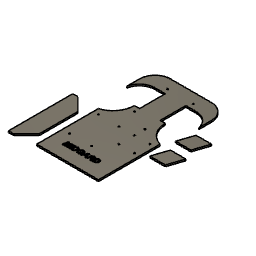
MIDGARD 3d (Autodesk Fusion 360 design; units mm, degrees)
Autodesk Fusion 360 part; units mm, degrees
note: some values were not read from the file. Chosen so that the rebuilt part matches the saved one: which bodies a step acts on.
sketch "Sketch1" plane through (0, 0, 0) normal (0, 1, 0) x (1, 0, 0)
  line L0 (60, 0) -> (60, -120)
  line L1 (60, -120) -> (-60, -120)
  line L2 (-60, -120) -> (-60, 0)
  line L3 (20, 40) -> (20, 90)
  line L4 (-20, 90) -> (-20, 40)
  line L5 (40, 120) -> (-40, 120)
  arc A0 (-40, 120) -> (-70, 90) centre (-40, 90) ccw
  line L6 (-70, 90) -> (-70, 65)
  arc A1 (-40, 90) -> (-70, 65) centre (-40, 59.5) ccw
  arc A2 (70, 90) -> (40, 120) centre (40, 90) ccw
  line L7 (70, 90) -> (70, 65)
  arc A3 (70, 65) -> (70, 66.4639) centre (45.1933, 65.732) ccw
  arc A4 (-60, 0) -> (-30, 40) centre (-71.6667, 40) ccw
  arc A5 (30, 40) -> (60, 0) centre (71.6667, 40) ccw
  arc A6 (70, 65) -> (40, 90) centre (40, 59.5) ccw
  line L8 (30, 40) -> (20, 40)
  line L9 (-20, 40) -> (-30, 40)
  line L10 (-40, 90) -> (-20, 90)
  line L11 (20, 90) -> (40, 90)
  line L12 (-75, -100) -> (-75, -25)
  line L13 (-100, 0) -> (-75, -25)
  line L14 (-75, -100) -> (-100, -125)
  line L15 (80, 50) -> (110, 50)
  line L16 (110, 50) -> (100, 20)
  line L17 (100, 20) -> (70, 20)
  line L18 (70, 20) -> (80, 50)
  line L19 (80, 0) -> (110, 0)
  line L20 (110, 0) -> (100, -30)
  line L21 (70, -30) -> (80, 0)
  line L22 (100, -30) -> (70, -30)
  line L23 (-110, 0) -> (-100, 0)
  line L24 (-100, -125) -> (-110, -125)
  line L25 (-110, -125) -> (-110, 0)
  line L26 (-26.9347, -100.4858) -> (-28.8856, -100.4758)
  line L27 (-28.8856, -100.4758) -> (-29.2041, -92.1179)
  line L28 (-29.2041, -92.1179) -> (-30.8365, -100.4657)
  line L29 (-30.8365, -100.4657) -> (-32.6918, -100.4562)
  line L30 (-32.6918, -100.4562) -> (-30.5531, -90.467)
  line L31 (-30.5531, -90.467) -> (-27.6199, -90.4821)
  line L32 (-27.6199, -90.4821) -> (-27.3491, -97.4891)
  line L33 (-27.3491, -97.4891) -> (-23.9024, -90.5013)
  line L34 (-23.9024, -90.5013) -> (-20.9352, -90.5166)
  line L35 (-20.9352, -90.5166) -> (-23.0808, -100.5056)
  line L36 (-23.0808, -100.5056) -> (-24.9566, -100.496)
  line L37 (-24.9566, -100.496) -> (-22.9426, -92.2116)
  line L38 (-22.9426, -92.2116) -> (-26.9347, -100.4858)
  line L39 (-21.1367, -100.5157) -> (-18.9911, -90.5266)
  line L40 (-18.9911, -90.5266) -> (-16.938, -90.5371)
  line L41 (-16.938, -90.5371) -> (-19.0767, -100.5263)
  line L42 (-19.0767, -100.5263) -> (-21.1367, -100.5157)
  line L43 (-17.1327, -100.5363) -> (-14.9871, -90.5472)
  line L44 (-14.9871, -90.5472) -> (-12.2927, -90.5611)
  spline S0 degree 2 poles (-12.2927, -90.5611) (-11.1672, -90.5669) (-10.8536, -90.6026) knots 0 0 0 1 1 1
  spline S1 degree 2 poles (-10.8536, -90.6026) (-10.2332, -90.6672) (-9.7465, -90.8607) knots 0 0 0 1 1 1
  spline S2 degree 2 poles (-9.7465, -90.8607) (-9.2598, -91.0542) (-8.8625, -91.4007) knots 0 0 0 1 1 1
  spline S3 degree 2 poles (-8.8625, -91.4007) (-8.4652, -91.7472) (-8.1778, -92.233) knots 0 0 0 1 1 1
  spline S4 degree 2 poles (-8.1778, -92.233) (-7.8904, -92.7188) (-7.7368, -93.3506) knots 0 0 0 1 1 1
  spline S5 degree 2 poles (-7.7368, -93.3506) (-7.5831, -93.9824) (-7.587, -94.7327) knots 0 0 0 1 1 1
  spline S6 degree 2 poles (-7.587, -94.7327) (-7.5953, -96.3493) (-8.2191, -97.5978) knots 0 0 0 1 1 1
  spline S7 degree 2 poles (-8.2191, -97.5978) (-8.8428, -98.8463) (-9.7811, -99.5782) knots 0 0 0 1 1 1
  spline S8 degree 2 poles (-9.7811, -99.5782) (-10.5003, -100.1475) (-11.634, -100.4145) knots 0 0 0 1 1 1
  spline S9 degree 2 poles (-11.634, -100.4145) (-12.276, -100.5613) (-13.6061, -100.5544) knots 0 0 0 1 1 1
  line L45 (-13.6061, -100.5544) -> (-17.1327, -100.5363)
  line L46 (-14.7302, -98.9388) -> (-13.6865, -98.9442)
  spline S10 degree 2 poles (-13.6865, -98.9442) (-12.5542, -98.95) (-12.0453, -98.8128) knots 0 0 0 1 1 1
  spline S11 degree 2 poles (-12.0453, -98.8128) (-11.5364, -98.6756) (-11.1115, -98.2958) knots 0 0 0 1 1 1
  spline S12 degree 2 poles (-11.1115, -98.2958) (-10.5016, -97.7464) (-10.0808, -96.8277) knots 0 0 0 1 1 1
  spline S13 degree 2 poles (-10.0808, -96.8277) (-9.6599, -95.9089) (-9.6535, -94.6607) knots 0 0 0 1 1 1
  spline S14 degree 2 poles (-9.6535, -94.6607) (-9.648, -93.5966) (-9.9897, -93.0593) knots 0 0 0 1 1 1
  spline S15 degree 2 poles (-9.9897, -93.0593) (-10.3314, -92.5221) (-10.8353, -92.3421) knots 0 0 0 1 1 1
  spline S16 degree 2 poles (-10.8353, -92.3421) (-11.1894, -92.2175) (-12.0966, -92.2128) knots 0 0 0 1 1 1
  line L47 (-12.0966, -92.2128) -> (-13.2903, -92.2067)
  line L48 (-13.2903, -92.2067) -> (-14.7302, -98.9388)
  line L49 (-1.4847, -95.2757) -> (2.99, -95.2988)
  line L50 (2.99, -95.2988) -> (2.0675, -99.5847)
  spline S17 degree 2 poles (2.0675, -99.5847) (1.2737, -100.0922) (0.1225, -100.4409) knots 0 0 0 1 1 1
  spline S18 degree 2 poles (0.1225, -100.4409) (-1.0287, -100.7897) (-2.2224, -100.7836) knots 0 0 0 1 1 1
  spline S19 degree 2 poles (-2.2224, -100.7836) (-4.0778, -100.774) (-5.0626, -99.9299) knots 0 0 0 1 1 1
  spline S20 degree 2 poles (-5.0626, -99.9299) (-6.4073, -98.777) (-6.3961, -96.6011) knots 0 0 0 1 1 1
  spline S21 degree 2 poles (-6.3961, -96.6011) (-6.3885, -95.1413) (-5.8018, -93.8074) knots 0 0 0 1 1 1
  spline S22 degree 2 poles (-5.8018, -93.8074) (-5.0978, -92.2011) (-3.8108, -91.321) knots 0 0 0 1 1 1
  spline S23 degree 2 poles (-3.8108, -91.321) (-2.5239, -90.4408) (-0.7913, -90.4498) knots 0 0 0 1 1 1
  spline S24 degree 2 poles (-0.7913, -90.4498) (0.9413, -90.4587) (1.9842, -91.269) knots 0 0 0 1 1 1
  spline S25 degree 2 poles (1.9842, -91.269) (3.0271, -92.0793) (3.3602, -93.6226) knots 0 0 0 1 1 1
  line L51 (3.3602, -93.6226) -> (1.4423, -93.831)
  spline S26 degree 2 poles (1.4423, -93.831) (1.1943, -92.9839) (0.6338, -92.5513) knots 0 0 0 1 1 1
  spline S27 degree 2 poles (0.6338, -92.5513) (0.0732, -92.1186) (-0.7794, -92.1142) knots 0 0 0 1 1 1
  spline S28 degree 2 poles (-0.7794, -92.1142) (-1.7753, -92.1091) (-2.6102, -92.6232) knots 0 0 0 1 1 1
  spline S29 degree 2 poles (-2.6102, -92.6232) (-3.445, -93.1374) (-3.9213, -94.2195) knots 0 0 0 1 1 1
  spline S30 degree 2 poles (-3.9213, -94.2195) (-4.3975, -95.3016) (-4.4041, -96.584) knots 0 0 0 1 1 1
  spline S31 degree 2 poles (-4.4041, -96.584) (-4.4106, -97.8459) (-3.8408, -98.4526) knots 0 0 0 1 1 1
  spline S32 degree 2 poles (-3.8408, -98.4526) (-3.2709, -99.0592) (-2.1658, -99.0649) knots 0 0 0 1 1 1
  spline S33 degree 2 poles (-2.1658, -99.0649) (-1.5042, -99.0683) (-0.8075, -98.8843) knots 0 0 0 1 1 1
  spline S34 degree 2 poles (-0.8075, -98.8843) (-0.1107, -98.7003) (0.3954, -98.4437) knots 0 0 0 1 1 1
  line L52 (0.3954, -98.4437) -> (0.71, -96.9583)
  line L53 (0.71, -96.9583) -> (-1.8411, -96.9451)
  line L54 (-1.8411, -96.9451) -> (-1.4847, -95.2757)
  line L55 (10.3476, -98.4677) -> (6.3845, -98.4472)
  line L56 (6.3845, -98.4472) -> (5.1726, -100.6511)
  line L57 (5.1726, -100.6511) -> (3.058, -100.6402)
  line L58 (3.058, -100.6402) -> (8.7643, -90.6695)
  line L59 (8.7643, -90.6695) -> (11.0494, -90.6813)
  line L60 (11.0494, -90.6813) -> (12.6213, -100.6895)
  line L61 (12.6213, -100.6895) -> (10.6705, -100.6794)
  line L62 (10.6705, -100.6794) -> (10.3476, -98.4677)
  line L63 (10.1038, -96.802) -> (9.5447, -92.7745)
  line L64 (9.5447, -92.7745) -> (7.1093, -96.7866)
  line L65 (7.1093, -96.7866) -> (10.1038, -96.802)
  line L66 (15.9774, -100.7068) -> (13.9174, -100.6962)
  line L67 (13.9174, -100.6962) -> (16.063, -90.7071)
  line L68 (16.063, -90.7071) -> (20.5036, -90.7299)
  spline S35 degree 2 poles (20.5036, -90.7299) (21.6495, -90.7358) (22.2861, -90.9745) knots 0 0 0 1 1 1
  spline S36 degree 2 poles (22.2861, -90.9745) (22.9227, -91.2131) (23.3117, -91.8426) knots 0 0 0 1 1 1
  spline S37 degree 2 poles (23.3117, -91.8426) (23.7006, -92.4722) (23.696, -93.3658) knots 0 0 0 1 1 1
  spline S38 degree 2 poles (23.696, -93.3658) (23.6895, -94.6414) (22.9212, -95.4662) knots 0 0 0 1 1 1
  spline S39 degree 2 poles (22.9212, -95.4662) (22.153, -96.291) (20.6036, -96.4809) knots 0 0 0 1 1 1
  spline S40 degree 2 poles (20.6036, -96.4809) (20.9974, -96.8376) (21.3423, -97.4192) knots 0 0 0 1 1 1
  spline S41 degree 2 poles (21.3423, -97.4192) (22.0252, -98.596) (22.86, -100.7422) knots 0 0 0 1 1 1
  line L69 (22.86, -100.7422) -> (20.6499, -100.7308)
  spline S42 degree 2 poles (20.6499, -100.7308) (20.3882, -99.8836) (19.6198, -98.0857) knots 0 0 0 1 1 1
  spline S43 degree 2 poles (19.6198, -98.0857) (19.2019, -97.1149) (18.7262, -96.7782) knots 0 0 0 1 1 1
  spline S44 degree 2 poles (18.7262, -96.7782) (18.4339, -96.5788) (17.704, -96.5751) knots 0 0 0 1 1 1
  line L70 (17.704, -96.5751) -> (16.865, -96.5708)
  line L71 (16.865, -96.5708) -> (15.9774, -100.7068)
  line L72 (17.1865, -95.0717) -> (18.2779, -95.0773)
  spline S45 degree 2 poles (18.2779, -95.0773) (19.9354, -95.0859) (20.4787, -94.8909) knots 0 0 0 1 1 1
  spline S46 degree 2 poles (20.4787, -94.8909) (21.022, -94.6958) (21.3312, -94.2745) knots 0 0 0 1 1 1
  spline S47 degree 2 poles (21.3312, -94.2745) (21.6403, -93.8532) (21.6427, -93.3893) knots 0 0 0 1 1 1
  spline S48 degree 2 poles (21.6427, -93.3893) (21.6455, -92.8436) (21.2035, -92.5685) knots 0 0 0 1 1 1
  spline S49 degree 2 poles (21.2035, -92.5685) (20.9315, -92.4034) (20.0243, -92.3987) knots 0 0 0 1 1 1
  line L73 (20.0243, -92.3987) -> (17.7597, -92.3871)
  line L74 (17.7597, -92.3871) -> (17.1865, -95.0717)
  line L75 (23.9991, -100.7481) -> (26.1447, -90.759)
  line L76 (26.1447, -90.759) -> (28.8391, -90.7729)
  spline S50 degree 2 poles (28.8391, -90.7729) (29.9646, -90.7787) (30.2782, -90.8144) knots 0 0 0 1 1 1
  spline S51 degree 2 poles (30.2782, -90.8144) (30.8986, -90.879) (31.3853, -91.0725) knots 0 0 0 1 1 1
  spline S52 degree 2 poles (31.3853, -91.0725) (31.872, -91.266) (32.2693, -91.6125) knots 0 0 0 1 1 1
  spline S53 degree 2 poles (32.2693, -91.6125) (32.6666, -91.959) (32.954, -92.4448) knots 0 0 0 1 1 1
  spline S54 degree 2 poles (32.954, -92.4448) (33.2414, -92.9306) (33.395, -93.5624) knots 0 0 0 1 1 1
  spline S55 degree 2 poles (33.395, -93.5624) (33.5487, -94.1942) (33.5448, -94.9445) knots 0 0 0 1 1 1
  spline S56 degree 2 poles (33.5448, -94.9445) (33.5365, -96.5611) (32.9127, -97.8096) knots 0 0 0 1 1 1
  spline S57 degree 2 poles (32.9127, -97.8096) (32.2889, -99.0581) (31.3506, -99.79) knots 0 0 0 1 1 1
  spline S58 degree 2 poles (31.3506, -99.79) (30.6315, -100.3593) (29.4978, -100.6263) knots 0 0 0 1 1 1
  spline S59 degree 2 poles (29.4978, -100.6263) (28.8558, -100.7731) (27.5257, -100.7662) knots 0 0 0 1 1 1
  line L77 (27.5257, -100.7662) -> (23.9991, -100.7481)
  line L78 (26.4016, -99.1506) -> (27.4453, -99.156)
  spline S60 degree 2 poles (27.4453, -99.156) (28.5776, -99.1618) (29.0865, -99.0246) knots 0 0 0 1 1 1
  spline S61 degree 2 poles (29.0865, -99.0246) (29.5954, -98.8874) (30.0203, -98.5076) knots 0 0 0 1 1 1
  spline S62 degree 2 poles (30.0203, -98.5076) (30.6302, -97.9582) (31.051, -97.0395) knots 0 0 0 1 1 1
  spline S63 degree 2 poles (31.051, -97.0395) (31.4719, -96.1207) (31.4783, -94.8725) knots 0 0 0 1 1 1
  spline S64 degree 2 poles (31.4783, -94.8725) (31.4838, -93.8084) (31.1421, -93.2711) knots 0 0 0 1 1 1
  spline S65 degree 2 poles (31.1421, -93.2711) (30.8003, -92.7339) (30.2965, -92.5539) knots 0 0 0 1 1 1
  spline S66 degree 2 poles (30.2965, -92.5539) (29.9424, -92.4293) (29.0352, -92.4246) knots 0 0 0 1 1 1
  line L79 (29.0352, -92.4246) -> (27.8415, -92.4185)
  line L80 (27.8415, -92.4185) -> (26.4016, -99.1506)
  circle A7 centre (-25, 100) radius 1.5
  circle A8 centre (25, 100) radius 1.5
  circle A9 centre (-20, 30) radius 1.5
  circle A10 centre (20, 0) radius 1.5
  circle A11 centre (-50, -10) radius 1.5
  circle A12 centre (-10, -10) radius 1.5
  circle A13 centre (-46.0467, -60) radius 1.5
  circle A14 centre (-5.7563, -60.4944) radius 1.5
  circle A15 centre (20, -20) radius 1.5
  circle A16 centre (50, -20) radius 1.5
  circle A17 centre (20, -50) radius 1.5
  circle A18 centre (50, -50) radius 1.5
  point P0 (71.6667, -10)
  dimension "d2" = 3
  dimension "d3" = 3
  dimension "d4" = 3
  dimension "d5" = 3
  dimension "d6" = 3
  dimension "d7" = 3
  dimension "d8" = 3
  dimension "d9" = 3
  dimension "d10" = 3
  dimension "d11" = 3
  dimension "d12" = 3
  dimension "d13" = 3
  constraint vertical L0
  constraint horizontal L1
  constraint vertical L2
  constraint horizontal L8
  constraint vertical L3
  constraint vertical L4
  constraint coincident L4.end L8
  constraint horizontal L10
  constraint horizontal L5
  constraint tangent L5 A0
  constraint tangent A0 L6
  constraint tangent A1 L10
  constraint tangent L5 A2
  constraint tangent A2 L7
  constraint coincident L7 A3.end
  constraint tangent A6 L10
  constraint collinear L8 L9
  constraint collinear L10 L11
  constraint vertical L12
  constraint horizontal L15
  constraint parallel L15 L17
  constraint parallel L16 L18
  constraint horizontal L19
  constraint parallel L19 L22
  constraint parallel L20 L21
  constraint horizontal L23
  constraint horizontal L24
  constraint vertical L25
  measures "d2" diameter of A7
  measures "d3" diameter of A8
  measures "d4" diameter of A9
  measures "d5" diameter of A10
  measures "d6" diameter of A11
  measures "d7" diameter of A12
  measures "d8" diameter of A13
  measures "d9" diameter of A14
  measures "d10" diameter of A15
  measures "d11" diameter of A16
  measures "d12" diameter of A17
  measures "d13" diameter of A18
extrude "Extrude1" add sketch "Sketch1" along normal blind 3 contours L0 L1 L2 L3 L4 L5 A0 L6 A1 A2 L7 A4 A5 A6 L8 L9 L10 L11 | L7 A3 | L12 L13 L14 L23 L24 L25 | L15 L16 L17 L18 | L19 L20 L21 L22 | L26 L27 L28 L29 L30 L31 L32 L33 L34 L35 L36 L37 L38 | L39 L40 L41 L42 | L43 L44 S0 S1 S2 S3 S4 S5 S6 S7 S8 S9 L45 | L46 S10 S11 S12 S13 S14 S15 S16 L47 L48 | L49 L50 S17 S18 S19 S20 S21 S22 S23 S24 S25 L51 S26 S27 S28 S29 S30 S31 S32 S33 S34 L52 L53 L54 | L55 L56 L57 L58 L59 L60 L61 L62 | L63 L64 L65 | L66 L67 L68 S35 S36 S37 S38 S39 S40 S41 L69 S42 S43 S44 L70 L71 | L72 S45 S46 S47 S48 S49 L73 L74 | L75 L76 S50 S51 S52 S53 S54 S55 S56 S57 S58 S59 L77 | L78 S60 S61 S62 S63 S64 S65 S66 L79 L80 | A7 | A8 | A9 | A10 | A11 | A12 | A13 | A14 | A15 | A16 | A17 | A18 makes body 1 at (83.3333, 0, 20) makes body 2 at (-98.3333, 0, 50) makes body 3 at (83.3333, 0, -30) makes body 4 at (16.3964, 0, 78.3613)
sketch "Sketch2" plane through (0, 3, 0) normal (0, 1, 0) x (-1, 0, 0)
  line L0 (-30, -40) -> (-20, -40)
  line L1 (-20, -40) -> (-20, -90)
  line L2 (-20, -90) -> (-40, -90)
  arc A0 (-70, -65) -> (-40, -90) centre (-40, -59.5) ccw
  arc A1 (-70, -65) -> (-70, -66.4639) centre (-45.1933, -65.732) ccw
  line L3 (-70, -66.4639) -> (-70, -90)
  arc A2 (-70, -90) -> (-40, -120) centre (-40, -90) ccw
  line L4 (-40, -120) -> (40, -120)
  arc A3 (40, -120) -> (70, -90) centre (40, -90) ccw
  line L5 (70, -90) -> (70, -65)
  arc A4 (40, -90) -> (70, -65) centre (40, -59.5) ccw
  line L6 (40, -90) -> (20, -90)
  line L7 (20, -90) -> (20, -40)
  line L8 (20, -40) -> (30, -40)
  arc A5 (60, 0) -> (30, -40) centre (71.6667, -40) ccw
  line L9 (60, 0) -> (60, 120)
  line L10 (60, 120) -> (-60, 120)
  line L11 (-60, 120) -> (-60, 0)
  arc A6 (-30, -40) -> (-60, 0) centre (-71.6667, -40) ccw
  line L12 (35.2213, 104.9214) -> (-36.3604, 103.98) construction
  line L13 (-36.3604, 103.98) -> (-36.104, 84.4836) construction
  line L14 (-36.104, 84.4836) -> (35.4777, 85.425) construction
  line L15 (35.4777, 85.425) -> (35.2213, 104.9214) construction
  dimension "d16" = 10
  text T0 "MIDGARD\n\n" font "Arial" height 10 bold italic align left top in box 71.5879 x 19.4981 at (35.2213, 104.9214) x (-0.999914, -0.01315) y (0.01315, -0.999914) spacing 1
extrude "Extrude2" cut sketch "Sketch2" against normal blind 3 text T0 bodies 4 makes body 5 at (-14.8696, 0, 90.6869) makes body 6 at (16.2624, 0, 87.3044) makes body 7 at (5.9555, 2, 88.3229) makes body 8 at (26.2592, 0, 90.146)
sketch "Sketch3" plane through (0, 3, 0) normal (0, 1, 0) x (-1, 0, 0)
  line L0 (19.7765, 85.2185) -> (21.7321, 95.2451)
  line L1 (21.7321, 95.2451) -> (23.792, 95.2722)
  line L2 (23.792, 95.2722) -> (21.8295, 85.2455)
  line L3 (21.8295, 85.2455) -> (19.7765, 85.2185)
  spline S0 degree 3 poles (-26.8361, 94.4563) (-26.566, 94.5033) (-25.915, 94.6166) (-25.2538, 94.6265) (-24.8669, 94.6322) knots 0 0 0 0 0.082119 0.197971 0.197971 0.197971 0.197971
  line L4 (-24.8669, 94.6322) -> (-21.3406, 94.6786)
  line L5 (-21.3406, 94.6786) -> (-23.303, 84.6519)
  line L6 (-23.303, 84.6519) -> (-25.9972, 84.6165)
  spline S1 degree 3 poles (-25.9972, 84.6165) (-26.3048, 84.6113) (-26.7849, 84.6033) (-27.2645, 84.6242) (-27.4368, 84.6317) knots 0 0 0 0 0.092262 0.143996 0.143996 0.143996 0.143996
  spline S2 degree 3 poles (-27.4368, 84.6317) (-27.6345, 84.6534) (-28.0132, 84.6951) (-28.3754, 84.8131) (-28.5485, 84.8695) knots 0 0 0 0 0.059492 0.11395 0.11395 0.11395 0.11395
  spline S3 degree 3 poles (-28.5485, 84.8695) (-28.7084, 84.9375) (-29.0287, 85.0739) (-29.3042, 85.2867) (-29.4422, 85.3932) knots 0 0 0 0 0.051899 0.103968 0.103968 0.103968 0.103968
  spline S4 degree 3 poles (-29.4422, 85.3932) (-29.5731, 85.5135) (-29.8395, 85.7584) (-30.04, 86.0596) (-30.142, 86.2129) knots 0 0 0 0 0.05312 0.108123 0.108123 0.108123 0.108123
  spline S5 degree 3 poles (-30.142, 86.2129) (-30.2362, 86.3827) (-30.4316, 86.7351) (-30.5448, 87.1219) (-30.6034, 87.3222) knots 0 0 0 0 0.058076 0.120474 0.120474 0.120474 0.120474
  spline S6 degree 3 poles (-30.6034, 87.3222) (-30.652, 87.5411) (-30.7529, 87.9953) (-30.7697, 88.4604) (-30.7785, 88.7013) knots 0 0 0 0 0.067121 0.139277 0.139277 0.139277 0.139277
  spline S7 degree 3 poles (-30.7785, 88.7013) (-30.7637, 89.2166) (-30.7352, 90.2093) (-30.3731, 91.1332) (-30.1989, 91.5775) knots 0 0 0 0 0.15332 0.295371 0.295371 0.295371 0.295371
  spline S8 degree 3 poles (-30.1989, 91.5775) (-29.992, 91.9705) (-29.5946, 92.7252) (-28.9719, 93.3072) (-28.6733, 93.5862) knots 0 0 0 0 0.132148 0.25382 0.25382 0.25382 0.25382
  spline S9 degree 3 poles (-28.6733, 93.5862) (-28.4093, 93.7705) (-27.8464, 94.1635) (-27.1864, 94.3547) (-26.8361, 94.4563) knots 0 0 0 0 0.095957 0.204513 0.204513 0.204513 0.204513
  line L7 (-9.9636, 94.8282) -> (-8.0129, 94.8539)
  line L8 (-8.0129, 94.8539) -> (-7.6496, 92.6484)
  line L9 (-7.6496, 92.6484) -> (-3.6868, 92.7005)
  line L10 (-3.6868, 92.7005) -> (-2.5154, 94.9262)
  line L11 (-2.5154, 94.9262) -> (-0.401, 94.954)
  line L12 (-0.401, 94.954) -> (-5.9239, 84.8805)
  line L13 (-5.9239, 84.8805) -> (-8.2088, 84.8504)
  line L14 (-8.2088, 84.8504) -> (-9.9636, 94.8282)
  line L15 (-14.9701, 90.6215) -> (-14.1312, 90.6325)
  line L16 (-14.1312, 90.6325) -> (-13.3194, 94.7841)
  line L17 (-13.3194, 94.7841) -> (-11.2596, 94.8112)
  line L18 (-11.2596, 94.8112) -> (-13.222, 84.7845)
  line L19 (-13.222, 84.7845) -> (-17.6623, 84.7261)
  spline S10 degree 3 poles (-17.6623, 84.7261) (-18.0042, 84.7252) (-18.6092, 84.7234) (-19.1945, 84.873) (-19.449, 84.938) knots 0 0 0 0 0.102063 0.180557 0.180557 0.180557 0.180557
  spline S11 degree 3 poles (-19.449, 84.938) (-19.654, 85.0324) (-20.0738, 85.2257) (-20.3493, 85.5972) (-20.4903, 85.7872) knots 0 0 0 0 0.066587 0.136311 0.136311 0.136311 0.136311
  spline S12 degree 3 poles (-20.4903, 85.7872) (-20.6076, 86.0128) (-20.8545, 86.4874) (-20.8859, 87.0223) (-20.9025, 87.3031) knots 0 0 0 0 0.075383 0.15867 0.15867 0.15867 0.15867
  spline S13 degree 3 poles (-20.9025, 87.3031) (-20.8805, 87.7049) (-20.8381, 88.4818) (-20.385, 89.1127) (-20.1662, 89.4173) knots 0 0 0 0 0.117945 0.228073 0.228073 0.228073 0.228073
  spline S14 degree 3 poles (-20.1662, 89.4173) (-19.8626, 89.6734) (-19.1967, 90.2351) (-18.3359, 90.39) (-17.8675, 90.4743) knots 0 0 0 0 0.117136 0.256964 0.256964 0.256964 0.256964
  spline S15 degree 3 poles (-17.8675, 90.4743) (-18.0022, 90.6054) (-18.2892, 90.8847) (-18.5075, 91.2207) (-18.6232, 91.3989) knots 0 0 0 0 0.056226 0.119752 0.119752 0.119752 0.119752
  spline S16 degree 3 poles (-18.6232, 91.3989) (-18.8798, 91.8638) (-19.469, 92.9314) (-19.9372, 94.0577) (-20.2015, 94.6936) knots 0 0 0 0 0.159174 0.365562 0.365562 0.365562 0.365562
  line L20 (-20.2015, 94.6936) -> (-17.9916, 94.7227)
  spline S17 degree 3 poles (-17.9916, 94.7227) (-17.8589, 94.3621) (-17.5319, 93.4736) (-17.1439, 92.6099) (-16.9133, 92.0968) knots 0 0 0 0 0.115231 0.283939 0.283939 0.283939 0.283939
  spline S18 degree 3 poles (-16.9133, 92.0968) (-16.7827, 91.815) (-16.5561, 91.326) (-16.1626, 90.9607) (-15.9958, 90.8059) knots 0 0 0 0 0.092018 0.159697 0.159697 0.159697 0.159697
  spline S19 degree 3 poles (-15.9958, 90.8059) (-15.8627, 90.7504) (-15.5361, 90.6144) (-15.1806, 90.6189) (-14.9701, 90.6215) knots 0 0 0 0 0.042893 0.105164 0.105164 0.105164 0.105164
  line L21 (2.014, 91.3156) -> (4.565, 91.3491)
  line L22 (4.565, 91.3491) -> (4.2391, 89.6735)
  line L23 (4.2391, 89.6735) -> (-0.2353, 89.6146)
  line L24 (-0.2353, 89.6146) -> (0.6086, 93.9167)
  spline S20 degree 3 poles (0.6086, 93.9167) (0.8956, 94.0877) (1.5073, 94.452) (2.1804, 94.6849) (2.5377, 94.8084) knots 0 0 0 0 0.099947 0.213017 0.213017 0.213017 0.213017
  spline S21 degree 3 poles (2.5377, 94.8084) (2.9209, 94.917) (3.6858, 95.1335) (4.4797, 95.1738) (4.8759, 95.1939) knots 0 0 0 0 0.119057 0.237653 0.237653 0.237653 0.237653
  spline S22 degree 3 poles (4.8759, 95.1939) (5.4383, 95.1821) (6.4637, 95.1606) (7.3369, 94.6313) (7.7312, 94.3924) knots 0 0 0 0 0.165218 0.301218 0.301218 0.301218 0.301218
  spline S23 degree 3 poles (7.7312, 94.3924) (8.1306, 93.9534) (8.9794, 93.0203) (9.0749, 91.7573) (9.1254, 91.0885) knots 0 0 0 0 0.173085 0.367882 0.367882 0.367882 0.367882
  spline S24 degree 3 poles (9.1254, 91.0885) (9.1076, 90.6068) (9.0721, 89.644) (8.7456, 88.7374) (8.5824, 88.2844) knots 0 0 0 0 0.143639 0.287153 0.287153 0.287153 0.287153
  spline S25 degree 3 poles (8.5824, 88.2844) (8.3397, 87.7796) (7.8689, 86.8006) (7.0392, 86.1009) (6.6372, 85.762) knots 0 0 0 0 0.165888 0.321758 0.321758 0.321758 0.321758
  spline S26 degree 3 poles (6.6372, 85.762) (6.1867, 85.4975) (5.2595, 84.953) (4.186, 84.8755) (3.6342, 84.8356) knots 0 0 0 0 0.154539 0.318054 0.318054 0.318054 0.318054
  spline S27 degree 3 poles (3.6342, 84.8356) (3.1, 84.8512) (2.1045, 84.8802) (1.2433, 85.3747) (0.8441, 85.6039) knots 0 0 0 0 0.157413 0.293394 0.293394 0.293394 0.293394
  spline S28 degree 3 poles (0.8441, 85.6039) (0.5181, 85.9102) (-0.1674, 86.5541) (-0.4346, 87.458) (-0.5747, 87.932) knots 0 0 0 0 0.131764 0.27704 0.27704 0.27704 0.27704
  line L25 (-0.5747, 87.932) -> (1.339, 88.1755)
  spline S29 degree 3 poles (1.339, 88.1755) (1.4333, 87.917) (1.6115, 87.4288) (1.9919, 87.0765) (2.1709, 86.9107) knots 0 0 0 0 0.08119 0.153321 0.153321 0.153321 0.153321
  spline S30 degree 3 poles (2.1709, 86.9107) (2.3787, 86.7882) (2.8162, 86.5302) (3.3248, 86.5101) (3.5918, 86.4996) knots 0 0 0 0 0.071232 0.149987 0.149987 0.149987 0.149987
  spline S31 degree 3 poles (3.5918, 86.4996) (3.9161, 86.5251) (4.5619, 86.5759) (5.13, 86.8871) (5.4129, 87.042) knots 0 0 0 0 0.096373 0.191952 0.191952 0.191952 0.191952
  spline S32 degree 3 poles (5.4129, 87.042) (5.676, 87.2502) (6.2299, 87.6884) (6.5346, 88.3269) (6.6946, 88.662) knots 0 0 0 0 0.099289 0.209021 0.209021 0.209021 0.209021
  spline S33 degree 3 poles (6.6946, 88.662) (6.8269, 89.0379) (7.0973, 89.8057) (7.1217, 90.6195) (7.1341, 91.035) knots 0 0 0 0 0.118771 0.242626 0.242626 0.242626 0.242626
  spline S34 degree 3 poles (7.1341, 91.035) (7.1182, 91.4128) (7.0898, 92.0912) (6.7065, 92.6468) (6.5366, 92.8929) knots 0 0 0 0 0.110668 0.198696 0.198696 0.198696 0.198696
  spline S35 degree 3 poles (6.5366, 92.8929) (6.3084, 93.0657) (5.8126, 93.4412) (5.188, 93.4628) (4.8508, 93.4745) knots 0 0 0 0 0.083871 0.182239 0.182239 0.182239 0.182239
  spline S36 degree 3 poles (4.8508, 93.4745) (4.6266, 93.4631) (4.1682, 93.4397) (3.7232, 93.3268) (3.496, 93.2691) knots 0 0 0 0 0.067183 0.137333 0.137333 0.137333 0.137333
  spline S37 degree 3 poles (3.496, 93.2691) (3.2786, 93.2036) (2.8684, 93.08) (2.4827, 92.894) (2.3014, 92.8065) knots 0 0 0 0 0.067982 0.128274 0.128274 0.128274 0.128274
  line L26 (2.3014, 92.8065) -> (2.014, 91.3156)
  spline S38 degree 3 poles (14.2927, 94.9972) (14.5628, 95.0442) (15.2138, 95.1575) (15.875, 95.1674) (16.2619, 95.1731) knots 0 0 0 0 0.082119 0.197971 0.197971 0.197971 0.197971
  line L27 (16.2619, 95.1731) -> (19.7882, 95.2195)
  line L28 (19.7882, 95.2195) -> (17.8258, 85.1928)
  line L29 (17.8258, 85.1928) -> (15.1316, 85.1574)
  spline S39 degree 3 poles (15.1316, 85.1574) (14.824, 85.1522) (14.3439, 85.1442) (13.8643, 85.1651) (13.692, 85.1726) knots 0 0 0 0 0.092262 0.143996 0.143996 0.143996 0.143996
  spline S40 degree 3 poles (13.692, 85.1726) (13.4943, 85.1943) (13.1155, 85.236) (12.7534, 85.354) (12.5803, 85.4104) knots 0 0 0 0 0.059492 0.11395 0.11395 0.11395 0.11395
  spline S41 degree 3 poles (12.5803, 85.4104) (12.4204, 85.4784) (12.1001, 85.6148) (11.8246, 85.8276) (11.6866, 85.9341) knots 0 0 0 0 0.051899 0.103968 0.103968 0.103968 0.103968
  spline S42 degree 3 poles (11.6866, 85.9341) (11.5557, 86.0544) (11.2893, 86.2993) (11.0888, 86.6005) (10.9868, 86.7538) knots 0 0 0 0 0.05312 0.108123 0.108123 0.108123 0.108123
  spline S43 degree 3 poles (10.9868, 86.7538) (10.8926, 86.9236) (10.6972, 87.276) (10.584, 87.6628) (10.5254, 87.8631) knots 0 0 0 0 0.058076 0.120474 0.120474 0.120474 0.120474
  spline S44 degree 3 poles (10.5254, 87.8631) (10.4767, 88.082) (10.3758, 88.5362) (10.359, 89.0013) (10.3503, 89.2422) knots 0 0 0 0 0.067121 0.139277 0.139277 0.139277 0.139277
  spline S45 degree 3 poles (10.3503, 89.2422) (10.3651, 89.7575) (10.3936, 90.7502) (10.7557, 91.6741) (10.9299, 92.1184) knots 0 0 0 0 0.15332 0.295371 0.295371 0.295371 0.295371
  spline S46 degree 3 poles (10.9299, 92.1184) (11.1368, 92.5114) (11.5342, 93.2661) (12.1569, 93.8481) (12.4554, 94.1271) knots 0 0 0 0 0.132148 0.25382 0.25382 0.25382 0.25382
  spline S47 degree 3 poles (12.4554, 94.1271) (12.7195, 94.3114) (13.2824, 94.7044) (13.9424, 94.8956) (14.2927, 94.9972) knots 0 0 0 0 0.095958 0.204514 0.204514 0.204514 0.204514
  line L30 (27.6116, 95.3224) -> (25.7495, 87.0025)
  line L31 (25.7495, 87.0025) -> (29.5896, 95.3484)
  line L32 (29.5896, 95.3484) -> (31.5403, 95.3741)
  line L33 (31.5403, 95.3741) -> (32.0117, 87.0235)
  line L34 (32.0117, 87.0235) -> (33.491, 95.3997)
  line L35 (33.491, 95.3997) -> (35.3462, 95.4241)
  line L36 (35.3462, 95.4241) -> (33.3906, 85.3975)
  line L37 (33.3906, 85.3975) -> (30.4577, 85.359)
  line L38 (30.4577, 85.359) -> (30.0586, 92.3598)
  line L39 (30.0586, 92.3598) -> (26.7404, 85.3101)
  line L40 (26.7404, 85.3101) -> (23.7734, 85.2711)
  line L41 (23.7734, 85.2711) -> (25.7359, 95.2977)
  line L42 (25.7359, 95.2977) -> (27.6116, 95.3224)
  line L43 (-30, -40) -> (-20, -40)
  line L44 (-20, -40) -> (-20, -90)
  line L45 (-20, -90) -> (-40, -90)
  arc A0 (-70, -65) -> (-40, -90) centre (-40, -59.5) ccw
  arc A1 (-70, -65) -> (-70, -66.4639) centre (-45.1933, -65.732) ccw
  line L46 (-70, -66.4639) -> (-70, -90)
  arc A2 (-70, -90) -> (-40, -120) centre (-40, -90) ccw
  line L47 (-40, -120) -> (40, -120)
  arc A3 (40, -120) -> (70, -90) centre (40, -90) ccw
  line L48 (70, -90) -> (70, -65)
  arc A4 (40, -90) -> (70, -65) centre (40, -59.5) ccw
  line L49 (40, -90) -> (20, -90)
  line L50 (20, -90) -> (20, -40)
  line L51 (20, -40) -> (30, -40)
  arc A5 (60, 0) -> (30, -40) centre (71.6667, -40) ccw
  line L52 (60, 0) -> (60, 120)
  line L53 (60, 120) -> (-60, 120)
  line L54 (-60, 120) -> (-60, 0)
  arc A6 (-30, -40) -> (-60, 0) centre (-71.6667, -40) ccw
  circle A7 centre (25.7359, -99.9687) radius 1.5
  circle A8 centre (-24.3943, -99.9687) radius 1.5
  circle A9 centre (20, -30) radius 1.5
  circle A10 centre (50, 10) radius 1.5
  circle A11 centre (10, 10) radius 1.5
  circle A12 centre (45.7361, 69.8145) radius 1.5
  circle A13 centre (3.5886, 69.4371) radius 1.5
  circle A14 centre (-20, 10) radius 1.5
  circle A15 centre (-50, 10) radius 1.5
  circle A16 centre (-20, 40) radius 1.5
  circle A17 centre (-50, 40) radius 1.5
  circle A18 centre (-20, -10) radius 1.5
  dimension "d19" = 3
  dimension "d20" = 3
  dimension "d21" = 3
  dimension "d23" = 3
  dimension "d24" = 3
  dimension "d25" = 3
  dimension "d26" = 3
  dimension "d27" = 3
  dimension "d28" = 3
  dimension "d29" = 3
  dimension "d30" = 3
  dimension "d31" = 3
  measures "d19" diameter of A7
  measures "d20" diameter of A8
  measures "d21" diameter of A9
  measures "d23" diameter of A10
  measures "d24" diameter of A11
  measures "d25" diameter of A12
  measures "d26" diameter of A13
  measures "d27" diameter of A14
  measures "d28" diameter of A15
  measures "d29" diameter of A16
  measures "d30" diameter of A17
  measures "d31" diameter of A18
extrude "Extrude3" cut sketch "Sketch3" against normal blind 3 contours A7 | A8 | A9 | A10 | A11 | A12 | A13 | A14 | A15 | A16 | A17 | A18 bodies 4
